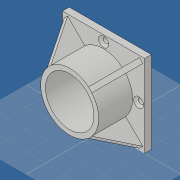
# Autodesk Inventor part: Zyklon_Flansch
Saved by Autodesk Inventor 2019 (Build 230136000, 136)
## iProperties
Created: 2020-08-01
Part Number: Zyklon_Flansch
Material: Generisch
Document SubType Name: Modeling
Designer: Stefan
Mass: 74.2474 g
Surface Area: 295.07 cm^2
Volume: 74.2474 cm^3
Density: 1 g/cm^3
Appearance: Vorgabe
Author: Stefan
Autodesk Inventor part; units mm, degrees
ref_plane "YZ Plane" through (0, 0, 0) normal (1, 0, 0) x (0, 1, 0)
ref_plane "XY Plane" through (0, 0, 0) normal (0, 0, 1) x (1, 0, 0)
sketch "Skizze1" plane through (0, 0, 0) normal (0, 0, 1) x (1, 0, 0)
  circle A0 centre (0, 0) radius 25.1
  circle A1 centre (0, 0) radius 30
  line L0 (-42.5, -42.5) -> (42.5, -42.5)
  line L1 (42.5, -42.5) -> (42.5, 42.5)
  line L2 (42.5, 42.5) -> (-42.5, 42.5)
  line L3 (-42.5, 42.5) -> (-42.5, -42.5)
  line L4 (-42.5, -42.5) -> (42.5, 42.5) construction
  line L5 (42.5, -42.5) -> (-42.5, 42.5) construction
  dimension "d0" = 50.2
  dimension "d2" = 60
  dimension "d25" = 85
  dimension "d26" = 85
  constraints: 12 end point, 3 midpoint, 2 centre point, 2 coincident, 2 parallel, 1 horizontal, 1 perpendicular
  measures "d0" diameter of A0
  measures "d2" diameter of A1
  measures "d25" distance of L2.end L1.end
  measures "d26" distance of L1.end L0.end
extrude "Extrusion1" add sketch "Skizze1" against normal blind 7 contours A1 | L3 L2 L1 L0
extrude "Extrusion2" add sketch "Skizze1" along normal blind 35 contours A1
ref_plane "Arbeitsebene1" through (0, 0, 0) normal (-0.7071, 0.7071, 0) x (0, 0, 1)
sketch "Skizze2" plane through (0, 0, 0) normal (-0.7071, 0.7071, 0) x (-0.7071, -0.7071, 0)
  line L0 (25.1, 35) -> (30, 35) projected
  line L1 (30, 35) -> (30, 0) projected
  line L2 (-30, 0) -> (-30, 35) projected
  line L3 (-30, 35) -> (-25.1, 35) projected
  line L4 (-30, 35) -> (-30, 0)
  line L5 (-30, 5) -> (-30, 35)
  line L6 (0, -15.4) -> (0, 43.4) projected
  line L7 (25.1, -7) -> (25.1, 35) projected
  line L8 (-25.1, 35) -> (-25.1, -7) projected
  line L9 (-60.1041, 0) -> (-30, 0) projected
  line L10 (30, 0) -> (60.1041, 0) projected
  line L11 (-60.1041, -7) -> (-60.1041, 0) projected
  line L12 (-25.1, -7) -> (-60.1041, -7) projected
  line L13 (60.1041, 0) -> (60.1041, -7) projected
  line L14 (60.1041, -7) -> (25.1, -7) projected
  line L15 (-30, 35) -> (-55, 0)
  line L16 (-30, 0) -> (-55, 0)
  line L17 (-30, 0) -> (-25.1, 0)
  line L18 (-25.1, 0) -> (-25.1, 35)
  line L19 (-25.1, 35) -> (-30, 35)
  line L20 (-30, 35) -> (-30, 0)
  point P0 (0, 0)
  point P1 (-42.5, -7)
  point P2 (0, 0)
  dimension "d28" = 25
  constraints: 16 end point, 2 collinear, 2 parallel, 1 horizontal, 1 perpendicular, 1 point on line
  measures "d28" distance of L2.start L15.end
extrude "Extrusion3" add sketch "Skizze2" along normal mid plane 5 contours L9 L15 L2 | L2 L3 L8 L17
pattern_circular "Runde Anordnung1" count 4 over 360 about axis through (0, 0, -10) along (0, 0, 1) of "Extrusion3"
sketch "Skizze3" plane through (0, 0, 0) normal (0, 0, 1) x (1, 0, 0)
  arc A0 (-19.3717, -22.9072) -> (19.3717, -22.9072) centre (0, 0) ccw projected
  arc A1 (-22.9072, 19.3717) -> (-22.9072, -19.3717) centre (0, 0) ccw projected
  arc A2 (22.9072, -19.3717) -> (22.9072, 19.3717) centre (0, 0) ccw projected
  line L0 (-42.5, 42.5) -> (-42.5, -42.5) projected
  circle A3 centre (0, 0) radius 42.5 construction
  circle A4 centre (0, 0) radius 30 construction
  circle A5 centre (0, 0) radius 36.25
  point P0 (-36.25, 0)
  dimension "d31" = 72.5
  dimension "d29" = 60
  dimension "d30" = 85
  constraints: 3 coincident, 2 centre point, 2 horizontal alignment, 2 tangent, 2 other
  measures "d29" diameter of A4
  measures "d30" diameter of A3
hole "Bohrung2" at (-36.25, 0, 0) direction (0, 0, -1) diameter 5.5 end through all countersink diameter 10.4 countersink angle 90 clearance for "Flachkopfsenkschraube DIN EN ISO 2009" size "M5" standard "DIN"
pattern_circular "Runde Anordnung3" count 4 over 360 about axis through (0, 0, -10) along (0, 0, 1) of "Bohrung2"
equation "\"d0\" = ht_diameter + 2 * gap_fit"
equation "\"kg_thickness\" = 4.9"
equation "\"ht_thickness\" = 1.9"
equation "\"case_thickness\" = 18"
equation "\"gap_fit\" = 0.1"
equation "\"gap_slide\" = 0.2"
equation "\"gap_air\" = 1"
equation "\"bore_diameter\" = 73"
equation "\"mdf_thickness\" = 6"
equation "\"tape_thickness\" = 3"
equation "\"tape_width\" = 15"
equation "\"inner_thickness\" = 15"
equation "\"inner_depth\" = 255"
equation "\"ht_diameter\" = 50"
